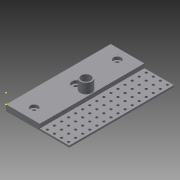
# Autodesk Inventor part: CraneBaseTest
Saved by Autodesk Inventor 2015 (Build 190159000, 159)
## iProperties
Created: 2016-03-19
Part Number: CraneBaseTest
Material: Generic
Document SubType Name: Modeling
Designer: Hatch
Density: 1 g/cm^3
Appearance: Default
Author: Hatch
Autodesk Inventor part; units mm, degrees
ref_plane "YZ Plane" through (0, 0, 0) normal (1, 0, 0) x (0, 1, 0)
ref_plane "XZ Plane" through (0, 0, 0) normal (0, 1, 0) x (-1, 0, 0)
ref_plane "XY Plane" through (0, 0, 0) normal (0, 0, 1) x (1, 0, 0)
sketch "Sketch1" plane through (0, 0, 0) normal (0, 1, 0) x (-1, 0, 0)
  line L0 (0, 0) -> (0, -177.8)
  line L1 (0, -177.8) -> (-57.15, -177.8)
  line L2 (0, 0) -> (-57.15, 0)
  line L3 (-57.15, 0) -> (-57.15, -177.8)
  dimension "d0" = 177.8
  dimension "d1" = 57.15
  constraints: 8 end point, 2 horizontal, 1 perpendicular, 1 vertical
  measures "d0" distance of L0.start L0.end
  measures "d1" distance of L0.end L1.end
extrude "Extrusion1" add sketch "Sketch1" along normal blind 10
sketch "Sketch2" plane through (0, 10, 0) normal (0, 1, 0) x (1, 0, 0)
  circle A0 centre (28.575, 88.9) radius 3.5
  point P0 (0, 0)
  dimension "d4" = 7
  constraints: 1 centre point
  measures "d4" diameter of A0
extrude "Extrusion2" cut sketch "Sketch2" against normal through all
pattern_linear "Rectangular Pattern1" count 2 spacing 71.4375 along (0, 0, -1) count 2 spacing 69.85 along (0, 0, 1) of "Extrusion2"
sketch "Sketch3" plane through (0, 10, 0) normal (0, 1, 0) x (1, 0, 0)
  arc A0 (25.1662, 89.6938) -> (31.9838, 89.6937) centre (28.575, 88.9) ccw projected
  circle A1 centre (28.575, 88.9) radius 6.5
  point P0 (0, 0)
  dimension "d13" = 13
  constraints: 1 centre point, 1 coincident
  measures "d13" diameter of A1
extrude "Extrusion3" cut sketch "Sketch3" against normal blind 5
pattern_linear "Rectangular Pattern2" count 2 spacing 71.4375 along (0, 0, -1) count 2 spacing 69.85 along (0, 0, 1) of "Extrusion3"
sketch "Sketch4" plane through (57.15, 0, 0) normal (1, 0, 0) x (0, 0, -1)
  line L0 (177.8, 0) -> (177.8, 10) projected
  line L1 (0, 0) -> (177.8, 0)
  line L2 (177.8, 0) -> (177.8, 3)
  line L3 (177.8, 3) -> (0, 3)
  line L4 (0, 3) -> (0, 0)
  dimension "d22" = 3
  constraints: 8 end point, 2 parallel, 1 horizontal, 1 perpendicular, 1 point on line
  measures "d22" distance of L2.end L1.end
extrude "Extrusion4" add sketch "Sketch4" along normal blind 50
sketch "Sketch5" plane through (57.15, 3, 0) normal (0, 1, 0) x (1, 0, 0)
  line L0 (50, 177.8) -> (50, 0) projected
  line L1 (0, 0) -> (0, 177.8) projected
  line L2 (0, 88.9) -> (8.125, 88.9)
  circle A0 centre (8.125, 88.9) radius 2.125
  point P0 (-57.15, 0)
  dimension "d25" = 8.125
  dimension "d26" = 4.25
  constraints: 2 end point, 1 centre point, 1 coincident, 1 midpoint
  measures "d25" distance of L2.start L2.end
  measures "d26" diameter of A0
extrude "Extrusion5" cut sketch "Sketch5" against normal through all
pattern_linear "Rectangular Pattern3" count 4 spacing 12 along (1, 0, 0) of "Extrusion5"
pattern_linear "Rectangular Pattern4" count 8 spacing 12 along (0, 0, 1) count 8 spacing 12 along (0, 0, -1) of "Extrusion5", "Rectangular Pattern3"
sketch "Sketch6" plane through (0, 10, 0) normal (0, 1, 0) x (1, 0, 0)
  arc A0 (25.1662, 89.6938) -> (31.9838, 89.6937) centre (28.575, 88.9) ccw projected
  line L0 (28.575, 85.4) -> (28.575, 93.9875)
  arc A1 (31.9838, 89.6937) -> (25.1662, 89.6938) centre (28.575, 90.4875) ccw projected
  line L1 (35.0264, 89.6938) -> (57.15, 89.6938)
  line L2 (57.15, 0) -> (57.15, 177.8) projected
  circle A2 centre (46.0882, 89.6938) radius 8
  circle A3 centre (46.0882, 89.6938) radius 10
  point P0 (0, 0)
  dimension "d38" = 16
  dimension "d39" = 20
  constraints: 4 end point, 2 centre point, 2 point on circle, 1 coincident, 1 horizontal, 1 midpoint, 1 point on line, 1 vertical
  measures "d38" diameter of A2
  measures "d39" diameter of A3
extrude "Extrusion6" add sketch "Sketch6" along normal blind 17 contours A2 L1 A3 | L1 A3 A2
sketch "Sketch7" plane through (46.0882, 10, -89.6938) normal (0, 1, 0) x (1, 0, 0)
  circle A0 centre (0, 0) radius 8 projected
  line L0 (-8, 0) -> (8, 0)
  point P0 (-46.0882, -89.6938)
  constraints: 2 end point, 2 point on circle, 1 horizontal
sketch "Sketch8" plane through (46.0882, 27, -89.6938) normal (0, 1, 0) x (1, 0, 0)
  point P0 (-46.0882, -89.6938)
body "Solid1"
